tappocamper (Autodesk Fusion 360 design; units mm, degrees)
Autodesk Fusion 360 part; units mm, degrees
sketch "Sketch1" plane through (0, 0, 0) normal (0, 0, 1) x (1, 0, 0)
  circle A0 centre (0, 0) radius 11.5
  circle A1 centre (0, 0) radius 14.5
  dimension "d1" = 23
  dimension "d2" = 29
  constraint coincident A0.centre A1.centre
  measures "d1" diameter of A0
  measures "d2" diameter of A1
extrude "Extrude1" add sketch "Sketch1" along normal blind 2.2 contours A0 | A1
extrude "Extrude2" add sketch "Sketch1" against normal blind 6 contours A0
fillet "Fillet1" radius 2 1 edges at (-13.5187, -5.2434, 2.2)
